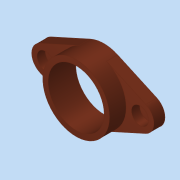
# Autodesk Inventor part: ShaftCollarMagnetMount
Saved by Autodesk Inventor 2017 (Build 210142000, 142)
## iProperties
Created: 2018-04-11
Part Number: ShaftCollarMagnetMount
Material: ABS Plastic
Document SubType Name: Modeling
Designer: Derek Wider
Density: 1.06 g/cm^3
Appearance: Copper - Satin
Author: Derek Wider
Autodesk Inventor part; units mm, degrees
ref_plane "YZ Plane" through (0, 0, 0) normal (1, 0, 0) x (0, 1, 0)
ref_plane "XZ Plane" through (0, 0, 0) normal (0, 1, 0) x (-1, 0, 0)
ref_plane "XY Plane" through (0, 0, 0) normal (0, 0, 1) x (1, 0, 0)
sketch "Sketch2" plane through (0, 0, 0) normal (0, 0, 1) x (1, 0, 0)
  circle A0 centre (0, 0) radius 5.05
  circle A1 centre (-8.5, 0) radius 1.55
  circle A2 centre (-8.5, 0) radius 2.5
  circle A3 centre (0, 0) radius 6
  line L0 (-2.4706, 5.4677) -> (-9.5294, 2.2782)
  line L1 (-9.5294, -2.2782) -> (-2.4706, -5.4677)
  circle A4 centre (8.5, 0) radius 1.55
  circle A5 centre (8.5, 0) radius 2.5
  line L2 (2.4706, 5.4677) -> (9.5294, 2.2782)
  line L3 (2.4706, -5.4677) -> (9.5294, -2.2782)
  dimension "d0" = 10.1
  dimension "d1" = 3.1
  dimension "d2" = 5
  dimension "d3" = 12
  constraints: 10 tangent, 8 end point, 8 point on circle, 6 centre point, 4 coincident, 2 equal radius
  measures "d0" diameter of A0
  measures "d1" diameter of A1
  measures "d2" diameter of A2
  measures "d3" diameter of A3
sketch "Sketch5" plane through (0, 0, 0) normal (0, 0, 1) x (1, 0, 0)
  circle A0 centre (0, 0) radius 6 projected
  circle A1 centre (0, 0) radius 5.05 projected
extrude "Extrusion5" add sketch "Sketch5" along normal blind 5
extrude "Extrusion6" add sketch "Sketch2" along normal blind 2 contours A0 | A2 | A3 L1 A2 | A2 L0 A3 | A3 | L2 A5 A3 | A3 A5 L3 | A5
sketch "Sketch6" plane through (0, 0, 2) normal (0, 0, 1) x (1, 0, 0)
  circle A0 centre (0, 0) radius 5.05 projected
extrude "Extrusion7" cut sketch "Sketch6" against normal through all
extrude "Extrusion8" add sketch "Sketch2" along normal blind 0.5 contours A1 | A4
body "Solid2"
